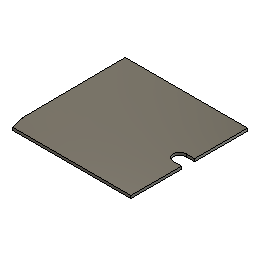
oceaan-25-floor_4 v2 (Autodesk Fusion 360 design; units mm, degrees)
Autodesk Fusion 360 part; units mm, degrees
note: some values were not read from the file. Set by a fixed rule: which sketch regions a step uses.
sketch "Sketch1" plane through (0, 0, 0) normal (0, 1, 0) x (1, 0, 0)
  line L0 (5, 0) -> (-542, 0)
  line L1 (5, 540) -> (-561, 540)
  line L2 (5, 540) -> (5, 295)
  line L3 (5, 540) -> (5, 295)
  line L4 (5, 295) -> (-33.6787, 295)
  line L5 (5, 235) -> (-33.6787, 235)
  line L6 (-557, 59.3636) -> (-542, 0)
  arc A0 (-33.6787, 295) -> (-33.6787, 235) centre (-33.6787, 265) ccw
  line L7 (5, 0) -> (5, 235)
  line L8 (5, 295) -> (5, 540)
  line L9 (-561, 540) -> (-557, 59.3636)
  dimension "d1" = 540
  dimension "d2" = 547
  dimension "d3" = 566
  dimension "d4" = 245
  dimension "d5" = 305
  dimension "d11" = 60
  dimension "d12" = 562
  constraint vertical L7
  constraint perpendicular L0 L7
  constraint perpendicular L1 L7
  constraint perpendicular L1 L2
  constraint perpendicular L1 L3
  constraint perpendicular L2 L4
  constraint perpendicular L5 L7
  constraint tangent L5 A0
  constraint collinear L7 L8
  measures "d1" distance of L0.start L1.start
  measures "d2" distance of L0.start L0.end
  measures "d3" distance of L1.start L1.end
  measures "d4" distance of L1.start L2.end
  measures "d5" distance of L1.start L5.start
  measures "d11" diameter of A0
  measures "d12" distance of L6.start L7
extrude "Extrude1" add sketch "Sketch1" along normal blind 12.5
equation "d3 = 562 mm + 4 mm"
